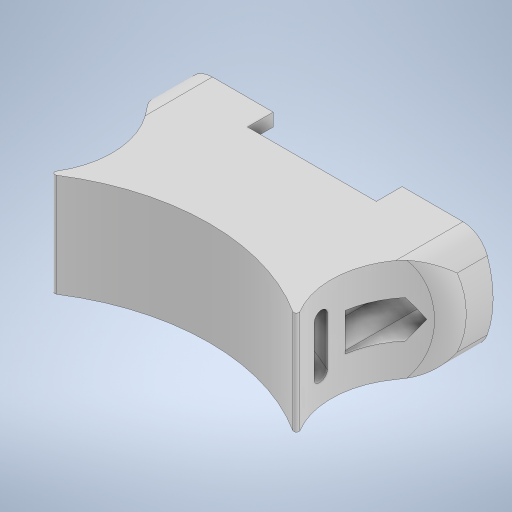
# Autodesk Inventor part: drzak_kable_spodni_dil_85_v2
Saved by Autodesk Inventor 2023 (Build 270158000, 158)
## iProperties
Created: 2025-01-22
Part Number: drzak_kable_spodni_dil_85_v2
Material: Všeobecné
Document SubType Name: Modeling
Designer: lisnik
Density: 1 g/cm^3
Appearance: Výchozí
Author: lisnik
Autodesk Inventor part; units mm, degrees
ref_plane "YZ Plane" through (0, 0, 0) normal (1, 0, 0) x (0, 1, 0)
ref_plane "XZ Plane" through (0, 0, 0) normal (0, 1, 0) x (-1, 0, 0)
ref_plane "XY Plane" through (0, 0, 0) normal (0, 0, 1) x (1, 0, 0)
sketch "Náčrt1" plane through (0, 0, 0) normal (0, 0, 1) x (1, 0, 0)
  line L0 (-24.5, 0) -> (24.5, 0) projected
  line L1 (0, -14) -> (0, 14) projected
  line L2 (-17.5, 10) -> (17.5, 10)
  line L3 (17.5, 10) -> (17.5, -10)
  line L4 (17.5, -10) -> (-17.5, -10)
  line L5 (-17.5, -10) -> (-17.5, 10)
  point P0 (0, 0)
  point P1 (0, 10)
  point P2 (17.5, 0)
  point P3 (-17.5, 0)
  point P4 (0, -10)
  dimension "d0" = 35
  dimension "d1" = 20
  constraints: 8 end point, 2 midpoint, 2 parallel, 2 point on line, 1 horizontal, 1 perpendicular
  measures "d0" distance of L3.end L4.end
  measures "d1" distance of L2.end L3.end
extrude "Vysunutí1" add sketch "Náčrt1" along normal blind 10
sketch "Náčrt2" plane through (0, 0, 0) normal (0, 0, -1) x (-1, 0, 0)
  line L0 (17.5, -10) -> (-17.5, -10) projected
  line L1 (17.5, 10) -> (17.5, -10) projected
  line L2 (-17.5, 10) -> (17.5, 10) projected
  line L3 (-17.5, -10) -> (-17.5, 10) projected
  line L4 (-15, 7.5) -> (15, 7.5)
  line L5 (15, 7.5) -> (15, -7.5)
  line L6 (15, -7.5) -> (-15, -7.5)
  line L7 (-15, -7.5) -> (-15, 7.5)
  line L8 (24.5, 0) -> (-24.5, 0) projected
  line L9 (0, -14) -> (0, 14) projected
  point P0 (0, 0)
  point P1 (0, 7.5)
  point P2 (15, 0)
  dimension "d4" = 15
  dimension "d5" = 30
  constraints: 8 end point, 2 midpoint, 2 parallel, 2 point on line, 1 horizontal, 1 perpendicular
  measures "d4" distance of L4.end L5.end
  measures "d5" distance of L4.start L4.end
extrude "Vysunutí2" cut sketch "Náčrt2" against normal blind 7.5 contours L9 L8 L5 L6 | L6 L7 L8 L9 | L8 L9 L4 L5 | L8 L7 L4 L9
sketch "Náčrt3" plane through (-17.5, 10, 0) normal (0, 1, 0) x (1, 0, 0)
  line L0 (35, 0) -> (0, 0) projected
  line L1 (0, 0) -> (0, -10) projected
  line L2 (35, -10) -> (0, -10) projected
  line L3 (35, 0) -> (35, -10) projected
  line L4 (30, -5) -> (5, -5)
  line L5 (5, -5) -> (5, 0)
  line L6 (5, 0) -> (30, 0)
  line L7 (30, 0) -> (30, -5)
  point P0 (17.5, 0)
  point P1 (17.5, 0)
  point P2 (30, 0)
  point P3 (5, 0)
  dimension "d8" = 5
  dimension "d9" = 25
  constraints: 8 end point, 2 midpoint, 2 parallel, 1 horizontal, 1 perpendicular
  measures "d8" distance of L4.end L5.end
  measures "d9" distance of L4.start L4.end
extrude "Vysunutí3" cut sketch "Náčrt3" against normal through all contours L7 L4 L5 L0
sketch "Náčrt4" plane through (0, 0, 0) normal (0, 0, -1) x (-1, 0, 0)
  line L0 (-12.5, 7.5) -> (-12.5, 10) projected
  line L1 (-17.5, 10) -> (-12.5, 10) projected
  line L2 (-17.5, -10) -> (-17.5, 10) projected
  line L3 (-12.5, -10) -> (-17.5, -10) projected
  line L4 (-12.5, -10) -> (-12.5, -7.5) projected
  line L5 (-12.5, -7.5) -> (-15, -7.5) projected
  line L6 (-15, -7.5) -> (-15, 7.5) projected
  line L7 (-15, 7.5) -> (-12.5, 7.5) projected
  line L8 (12.5, 10) -> (12.5, 7.5) projected
  line L9 (12.5, 7.5) -> (15, 7.5) projected
  line L10 (15, 7.5) -> (15, -7.5) projected
  line L11 (15, -7.5) -> (12.5, -7.5) projected
  line L12 (12.5, -7.5) -> (12.5, -10) projected
  line L13 (17.5, -10) -> (12.5, -10) projected
  line L14 (17.5, 10) -> (17.5, -10) projected
  line L15 (12.5, 10) -> (17.5, 10) projected
  line L16 (52.5, 0) -> (-52.5, 0) projected
  line L17 (0, -14) -> (0, 14) projected
  line L18 (-17.5, 10) -> (17.5, 10) projected
  line L19 (-27.5, 10) -> (-17.5, 10)
  line L20 (-17.5, 10) -> (-17.5, -10)
  line L21 (-17.5, -10) -> (-27.5, -10)
  line L22 (-27.5, -10) -> (-27.5, 10)
  line L23 (17.5, 10) -> (27.5, 10)
  line L24 (27.5, 10) -> (27.5, -10)
  line L25 (27.5, -10) -> (17.5, -10)
  line L26 (17.5, -10) -> (17.5, 10)
  arc A0 (-27.5, 10) -> (-27.5, -10) centre (-10, 0) ccw
  arc A1 (27.5, -10) -> (27.5, 10) centre (10, 0) ccw
  point P0 (0, 0)
  point P1 (-17.5, 0)
  point P2 (17.5, 0)
  point P3 (17.5, 0)
  point P4 (-17.5, 0)
  dimension "d37" = 10
  dimension "d38" = 10
  dimension "d99" = 10
  dimension "d100" = 10
  constraints: 16 end point, 5 midpoint, 5 point on line, 4 parallel, 4 point on circle, 2 centre point, 2 horizontal, 2 perpendicular
  measures "d37" distance of L23.start L23.end
  measures "d38" distance of L19.start L1.start
  measures "d99" distance from line of L17 A0.centre
  measures "d100" distance from line of L17 A1.centre
extrude "Vysunutí4" add sketch "Náčrt4" against normal blind 20 contours L2 L16 L22 L19 | L2 L21 L22 L16 | L22 L16 A0 | L22 A0 L16 | L23 L24 L16 L14 | L16 L24 L25 L14 | A1 L16 L24 | L16 A1 L24
sketch "Náčrt6" plane through (-17.5, 10, 10) normal (0, 1, 0) x (1, 0, 0)
  line L0 (30, 10) -> (30, 5) projected
  line L1 (30, 5) -> (5, 5) projected
  line L2 (5, 5) -> (5, 10) projected
  line L3 (5, 10) -> (-10, 10) projected
  line L4 (35, 0) -> (0, 0) projected
  line L5 (-10, 10) -> (-10, -10) projected
  line L6 (45, 10) -> (45, -10) projected
  line L7 (30, 10) -> (45, 10) projected
  line L8 (0, -10) -> (-10, -10) projected
  line L9 (0, 0) -> (0, -10) projected
  line L10 (35, 0) -> (35, -10) projected
  line L11 (45, -10) -> (35, -10) projected
  line L12 (17.5, 10) -> (17.5, -59.3976) construction
  line L13 (-10, 10) -> (-10, -10) projected
  line L14 (-10, 0) -> (45, 0)
  line L15 (45, 0) -> (45, -25)
  line L16 (45, -25) -> (-10, -25)
  line L17 (-10, -25) -> (-10, 0)
  arc A0 (45, -25) -> (-10, -25) centre (17.5, -57.4037) ccw
  point P0 (17.5, -14.9037)
  point P1 (17.5, 0)
  point P2 (-10, 0)
  point P3 (-10, -10)
  point P4 (45, -10)
  dimension "d59" = 42.5
  dimension "d60" = 25
  constraints: 10 end point, 3 midpoint, 3 point on circle, 2 parallel, 1 centre point, 1 coincident, 1 horizontal, 1 perpendicular, 1 vertical
  measures "d59" distance of A0.centre point (17.5, -14.904)
  measures "d60" distance of L14.end L15.end
extrude "Vysunutí5" add sketch "Náčrt6" against normal up to surface (20 mm away) contours L6 L11 L10 L14 | L15 A0 L17 L8 L9 L4 L10 L11 | L9 L8 L5 L14
sketch "Náčrt7" plane through (0, 0, 0) normal (1, 0, 0) x (0, 1, 0)
  line L0 (-9.8698, 24.9037) -> (10.1302, 24.9037)
  line L1 (-17.3035, 0) -> (33.8211, 0) projected
  line L2 (0, -12.746) -> (0, 76.4758) projected
  line L3 (6, 20.9037) -> (-6, 20.9037)
  line L4 (-6, 20.9037) -> (-6, 18.4037)
  line L5 (-6, 18.4037) -> (6, 18.4037)
  line L6 (6, 18.4037) -> (6, 20.9037)
  line L7 (0, 67.4037) -> (26.5176, 67.4037)
  line L8 (-10, 24.9037) -> (10, 24.9037) projected
  point P0 (0, 0)
  point P1 (0, 18.4037)
  point P2 (0, 24.9037)
  point P3 (0.1302, 24.9037)
  dimension "d30" = 42.5
  dimension "d31" = 2.5
  dimension "d32" = 4
  dimension "d33" = 6
  constraints: 12 end point, 4 point on line, 2 horizontal, 2 midpoint, 2 parallel, 1 perpendicular
  measures "d30" distance from line of L7.start L0
  measures "d31" distance of L5.end L3.start
  measures "d32" distance between parallel lines of L0 L3
  measures "d33" distance between parallel lines of L2 L6
revolve "Rotace1" cut sketch "Náčrt7" angle 360 about axis through (0, 0, 67.4037) along (0, -1, 0)
sketch "Náčrt10" plane through (0, 0, 0) normal (0, 0, -1) x (-1, 0, 0)
  line L0 (12.5, 10) -> (12.5, 7.5) projected
  line L1 (12.5, 7.5) -> (15, 7.5) projected
  line L2 (15, 7.5) -> (15, -7.5) projected
  line L3 (15, -7.5) -> (12.5, -7.5) projected
  line L4 (12.5, -7.5) -> (12.5, -10) projected
  line L5 (27.5, -10) -> (12.5, -10) projected
  arc A0 (27.5, -10) -> (27.5, 10) centre (10, 0) ccw projected
  line L6 (12.5, 10) -> (27.5, 10) projected
  line L7 (-12.5, 7.5) -> (-12.5, 10) projected
  line L8 (-12.5, 10) -> (-27.5, 10) projected
  arc A1 (-27.5, 10) -> (-27.5, -10) centre (-10, 0) ccw projected
  line L9 (-12.5, -10) -> (-27.5, -10) projected
  line L10 (-12.5, -10) -> (-12.5, -7.5) projected
  line L11 (-12.5, -7.5) -> (-15, -7.5) projected
  line L12 (-15, -7.5) -> (-15, 7.5) projected
  line L13 (-15, 7.5) -> (-12.5, 7.5) projected
  line L14 (42.2179, 0) -> (-42.2179, 0) projected
  line L15 (0, -14) -> (0, 14) projected
  circle A2 centre (23, 0) radius 2.25
  circle A3 centre (-23, 0) radius 2.25
  line L16 (18.7853, 0) -> (20.8927, 3.65)
  line L17 (20.8927, 3.65) -> (25.1073, 3.65)
  line L18 (25.1073, 3.65) -> (27.2147, 0)
  line L19 (27.2147, 0) -> (25.1073, -3.65)
  line L20 (25.1073, -3.65) -> (20.8927, -3.65)
  line L21 (20.8927, -3.65) -> (18.7853, 0)
  line L22 (-27.2147, 0) -> (-25.1073, 3.65)
  line L23 (-25.1073, 3.65) -> (-20.8927, 3.65)
  line L24 (-20.8927, 3.65) -> (-18.7853, 0)
  line L25 (-18.7853, 0) -> (-20.8927, -3.65)
  line L26 (-20.8927, -3.65) -> (-25.1073, -3.65)
  line L27 (-25.1073, -3.65) -> (-27.2147, 0)
  point P0 (0, 0)
  dimension "d61" = 46
  dimension "d62" = 23
  dimension "d63" = 4.5
  dimension "d64" = 4.5
  dimension "d65" = 3.65
  dimension "d66" = 3.65
  constraints: 24 end point, 4 coincident, 4 point on line, 2 centre point, 26 other
  measures "d61" distance of point (-23, 0) point (23, 0)
  measures "d62" distance from line of L15 point (-23, 0)
  measures "d63" diameter of A2
  measures "d64" diameter of A3
  measures "d65" distance between parallel lines of L14 L20
  measures "d66" distance between parallel lines of L14 L26
extrude "Vysunutí9" cut sketch "Náčrt10" against normal blind 20 contours A2 L14 | L14 A2 | A3 L14 | L14 A3
extrude "Vysunutí10" cut sketch "Náčrt10" along normal blind 15 from surface at -20 contours L19 L20 L21 L14 A2 | L14 A2 L16 L17 L18 | A2 L14 | L14 A2 | L25 L26 L27 L14 A3 | L14 A3 L22 L23 L24
sketch "Náčrt11" plane through (-12.5, -10, 5) normal (0, -1, 0) x (1, 0, 0)
  line L0 (25, 0) -> (25, -5) projected
  line L1 (25, -5) -> (40, -5) projected
  line L2 (40, -5) -> (40, 15) projected
  line L3 (40, 30) -> (40, 15) projected
  arc A0 (-15, 30) -> (40, 30) centre (12.5, 62.4037) ccw projected
  line L4 (-15, 15) -> (-15, 30) projected
  line L5 (-15, -5) -> (-15, 15) projected
  line L6 (-15, -5) -> (0, -5) projected
  line L7 (0, -5) -> (0, 0) projected
  line L8 (0, 0) -> (25, 0) projected
  line L9 (-15, -5) -> (-15, 15) projected
  line L10 (-15, 15) -> (-15, 15) projected
  line L11 (-15, -5) -> (-15, 15) projected
  line L12 (-15, -5) -> (-15, -5) projected
  circle A1 centre (50, 17.5) radius 16.25
  circle A2 centre (-25, 17.5) radius 16.25
  line L13 (-62.75, -5) -> (87.75, -5) projected
  line L14 (12.5, -18.4807) -> (12.5, 75.8844) projected
  point P0 (12.5, -5)
  dimension "d90" = 22.5
  dimension "d91" = 22.5
  dimension "d92" = 37.5
  dimension "d93" = 37.5
  dimension "d94" = 32.5
  dimension "d95" = 32.5
  constraints: 2 centre point, 1 other
  measures "d92" distance from line of A2.centre L14
  measures "d93" distance from line of L14 A1.centre
  measures "d94" diameter of A2
  measures "d95" diameter of A1
extrude "Vysunutí11" cut sketch "Náčrt11" against normal blind 25 contours A1 A0 L3 L2 | L2 L3 A0 A1 | A2 L5 L4 A0 | A0 L4 L5 A2
fillet "Zaoblení6" radius 0.5 2 edges at (25.3526, 0, 33.2936) (-25.3526, 0, 33.2936)
fillet "Zaoblení7" radius 1.25 4 edges at (0, 6, 18.4037) (0, 6, 20.9037) (0, -6, 20.9037) (0, -6, 18.4037)
fillet "Zaoblení9" radius 5 6 edges at (30.1556, 0.0032, 8.0044) (27.5, -10, 4.8457) (27.5, 10, 4.8457) (-27.5, -10, 4.8457) (-30.1556, 0.0033, 8.0044) (-27.5, 10, 4.8457)
